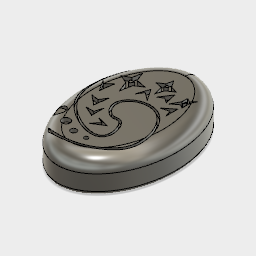
Heart of Te Fiti v12 (Autodesk Fusion 360 design; units mm, degrees)
Autodesk Fusion 360 part; units mm, degrees
sketch "Sketch1" plane through (0, 0, 0) normal (0, 1, 0) x (1, 0, 0)
  ellipse E0 centre (0, 0) end of major axis (-25.3296, 0) minor radius 36.9593
  line L0 (0, 36.9593) -> (0, -36.9593)
  spline S0 degree 5 poles (-15.7012, 29.002) (-15.9891, 28.3491) (-16.546, 27.0466) (-17.3246, 25.1025) (-18.2491, 22.5296) (-19.2149, 19.3463) (-19.9901, 16.1981) (-20.573, 13.0893) (-20.9615, 10.0271) (-21.1523, 7.0224) (-21.1416, 4.0904) (-20.9226, 1.2494) (-20.4826, -1.4829) (-19.7996, -4.0921) (-18.84, -6.57) (-17.5537, -8.9182) (-15.8765, -11.1484) (-13.7557, -13.2651) (-11.1725, -15.2534) (-8.1669, -17.0617) (-4.8575, -18.5914) (-1.4746, -19.6732) (1.6501, -20.0831) (4.1724, -19.6282) (5.8128, -18.2238) (6.4275, -15.9592) (6.1099, -13.2065) (5.1666, -10.5598) (3.9551, -8.5895) (2.7709, -7.6638) (1.6883, -7.7026) (0.4948, -8.076) (-1.034, -8.0508) (-2.8425, -7.2512) (-4.6232, -5.6824) (-5.9927, -3.5531) (-6.6094, -1.1715) (-6.3383, 1.2047) (-5.2263, 3.3819) (-3.4309, 5.2146) (-1.1685, 6.6006) (1.3532, 7.4698) (3.9703, 7.7796) (6.5518, 7.5146) (8.9989, 6.6859) (11.24, 5.3299) (13.2285, 3.5089) (14.9372, 1.306) (16.35, -1.1845) (17.4553, -3.8656) (18.2388, -6.6462) (18.6749, -9.4504) (18.7235, -12.2234) (18.3412, -14.9247) (17.4911, -17.5231) (16.1529, -19.9908) (14.3329, -22.2983) (12.0743, -24.4089) (9.4475, -26.2812) (6.5404, -27.8718) (3.4481, -29.1384) (0.2632, -30.0424) (-2.9336, -30.5517) (-6.0847, -30.6437) (-9.1516, -30.3038) (-12.1117, -29.5237) (-14.3851, -28.5443) (-16.0353, -27.6096) (-17.1111, -26.8975) (-17.6429, -26.5192) knots 0 0 0 0 0 0 0.01538462 0.03076923 0.04615385 0.06153846 0.07692308 0.09230769 0.10769231 0.12307692 0.13846154 0.15384615 0.16923077 0.18461538 0.2 0.21538462 0.23076923 0.24615385 0.26153846 0.27692308 0.29230769 0.30769231 0.32307692 0.33846154 0.35384615 0.36923077 0.38461538 0.4 0.41538462 0.43076923 0.44615385 0.46153846 0.47692308 0.49230769 0.50769231 0.52307692 0.53846154 0.55384615 0.56923077 0.58461538 0.6 0.61538462 0.63076923 0.64615385 0.66153846 0.67692308 0.69230769 0.70769231 0.72307692 0.73846154 0.75384615 0.76923077 0.78461538 0.8 0.81538462 0.83076923 0.84615385 0.86153846 0.87692308 0.89230769 0.90769231 0.92307692 0.93846154 0.95384615 0.96923077 0.98461538 1 1 1 1 1 1
  spline S1 degree 3 poles (-16.6162, 29.4055) (-19.4737, 22.9258) (-21.2452, 16.5844) (-21.871, 10.5048) (-22.3276, 6.0685) (-22.195, 1.7935) (-21.2955, -2.1346) (-20.5773, -5.2711) (-19.3583, -8.1903) (-17.2819, -10.8547) (-15.6727, -12.9195) (-13.5224, -14.8439) (-10.8813, -16.5273) (-8.5658, -18.0031) (-5.866, -19.3042) (-3.1892, -20.1044) (-0.8686, -20.7982) (1.4051, -21.1094) (3.2946, -20.663) (4.5251, -20.3723) (5.6026, -19.7124) (6.2825, -18.7299) (7.1836, -17.4276) (7.3498, -15.6939) (7.112, -14.0022) (6.8652, -12.2461) (6.209, -10.5186) (5.4431, -9.2339) (4.856, -8.2491) (4.2062, -7.505) (3.4287, -7.095) (2.8556, -6.7929) (2.2196, -6.7275) (1.7142, -6.7735) (0.9777, -6.8405) (0.4776, -7.0104) (-0.0835, -6.9994) (-0.6436, -6.9884) (-1.3083, -6.8203) (-2.0532, -6.3723) (-3.1341, -5.7222) (-4.2876, -4.4772) (-4.8945, -3.0786) (-5.5405, -1.5898) (-5.5712, -0.0001) (-4.9649, 1.4393) (-4.2274, 3.19) (-2.521, 4.7438) (-0.4724, 5.6612) (1.5863, 6.5831) (3.9224, 6.8611) (6.0735, 6.4445) (8.7058, 5.9347) (11.0949, 4.3826) (12.9846, 2.0916) (15.2894, -0.7024) (16.8696, -4.5298) (17.4301, -8.2498) (17.9455, -11.6702) (17.5729, -14.9779) (16.0429, -17.9581) (14.7902, -20.3981) (12.7277, -22.6602) (10.0863, -24.5365) (6.8505, -26.835) (2.8163, -28.5153) (-1.13, -29.199) (-4.8782, -29.8484) (-8.5276, -29.611) (-11.8947, -28.4189) (-13.6843, -27.7852) (-15.4056, -26.8835) (-17.0633, -25.7044) knots 0 0 0 0 0.09047855 0.09047855 0.09047855 0.15650286 0.15650286 0.15650286 0.20922143 0.20922143 0.20922143 0.25007582 0.25007582 0.25007582 0.28589274 0.28589274 0.28589274 0.3169454 0.3169454 0.3169454 0.3371678 0.3371678 0.3371678 0.36397047 0.36397047 0.36397047 0.39179297 0.39179297 0.39179297 0.41311949 0.41311949 0.41311949 0.42883763 0.42883763 0.42883763 0.45174167 0.45174167 0.45174167 0.47460508 0.47460508 0.47460508 0.50778137 0.50778137 0.50778137 0.54309603 0.54309603 0.54309603 0.58604666 0.58604666 0.58604666 0.62920969 0.62920969 0.62920969 0.68202832 0.68202832 0.68202832 0.7464456 0.7464456 0.7464456 0.80567522 0.80567522 0.80567522 0.85416995 0.85416995 0.85416995 0.91357908 0.91357908 0.91357908 0.97000737 0.97000737 0.97000737 1 1 1 1
  line L1 (-18.7775, -24.805) -> (-17.0633, -25.7044)
  line L2 (2, -13) -> (-3.7121, -16.5136)
  line L3 (-3.7121, -16.5136) -> (-0.856, -13)
  line L4 (-0.856, -13) -> (-3.7121, -11.6455)
  line L5 (-3.7121, -11.6455) -> (2, -13)
  line L6 (-6.8234, -12.3227) -> (-6.8234, -6)
  line L7 (-6.8234, -6) -> (-8, -10)
  line L8 (-8, -10) -> (-12, -10)
  line L9 (-12, -10) -> (-6.8234, -12.3227)
  line L10 (-16, -3) -> (-10.994, -7.0691)
  line L11 (-10.994, -7.0691) -> (-10, 0)
  line L12 (-10, 0) -> (-12.2593, -3.5345)
  line L13 (-12.2593, -3.5345) -> (-16, -3)
  line L14 (-20, 7) -> (-16, 1)
  line L15 (-16, 1) -> (-15, 8)
  line L16 (-15, 8) -> (-18, 5)
  line L17 (-18, 5) -> (-20, 7)
  line L18 (-17.1699, 13.2946) -> (-12.8176, 11.6267)
  line L19 (-12.8176, 11.6267) -> (-10.5661, 5.9978)
  line L20 (-10.5661, 5.9978) -> (-9.464, 11.8697)
  line L21 (-9.464, 11.8697) -> (-5.6699, 14.4447)
  line L22 (-5.6699, 14.4447) -> (-10.6699, 15.3832)
  line L23 (-10.6699, 15.3832) -> (-12.5397, 20.0577)
  line L24 (-12.5397, 20.0577) -> (-13.4171, 15.3832)
  line L25 (-13.4171, 15.3832) -> (-17.1699, 13.2946)
  line L26 (-12.9292, 13.9595) -> (-11.7996, 11.9649)
  line L27 (-11.7996, 11.9649) -> (-10.5246, 13.9595)
  line L28 (-10.5246, 13.9595) -> (-12.9292, 13.9595)
  line L29 (14.5337, 21.6256) -> (12.8041, 19.3149)
  line L30 (12.8041, 19.3149) -> (10.7477, 20.4148)
  line L31 (10.7477, 20.4148) -> (10.7477, 17.5434)
  line L32 (10.7477, 17.5434) -> (8.3775, 13.112)
  line L33 (8.3775, 13.112) -> (11.6761, 15.7091)
  line L34 (11.6761, 15.7091) -> (13.5759, 14.693)
  line L35 (13.5759, 14.693) -> (13.5759, 18.1878)
  line L36 (13.5759, 18.1878) -> (14.5337, 21.6256)
  line L37 (11.8441, 16.623) -> (12.6269, 18.0864)
  line L38 (12.6269, 18.0864) -> (11.8441, 18.5051)
  line L39 (11.8441, 18.5051) -> (11.8441, 16.623)
  line L40 (-5, 9) -> (-3, 15)
  line L41 (-3, 15) -> (1, 9)
  line L42 (1, 9) -> (-3, 12)
  line L43 (-3, 12) -> (-5, 9)
  line L44 (2, 13) -> (5.761, 18.6416)
  line L45 (5.761, 18.6416) -> (7, 13)
  line L46 (7, 13) -> (4.6288, 14.5808)
  line L47 (4.6288, 14.5808) -> (2, 13)
  line L48 (8, 9) -> (13, 13)
  line L49 (13, 13) -> (13, 7)
  line L50 (13, 7) -> (12, 10)
  line L51 (12, 10) -> (8, 9)
  line L52 (0, 14) -> (1.3214, 17.9641)
  line L53 (1.3214, 17.9641) -> (4.7927, 20.2783)
  line L54 (4.7927, 20.2783) -> (1.3214, 21.4354)
  line L55 (1.3214, 21.4354) -> (-0.8933, 24.7574)
  line L56 (-0.8933, 24.7574) -> (-1.5471, 21.4354)
  line L57 (-1.5471, 21.4354) -> (-4.7582, 19.2947)
  line L58 (-4.7582, 19.2947) -> (-1.2202, 18.5984)
  line L59 (-1.2202, 18.5984) -> (0, 14)
  line L60 (-0.6101, 21.4354) -> (0.6607, 20.3651)
  line L61 (0.6607, 20.3651) -> (-0.6101, 19.2947)
  line L62 (-0.6101, 19.2947) -> (-0.6101, 21.4354)
  circle A0 centre (-18.5, -17.5) radius 2.9155
  circle A1 centre (-11, -21.5) radius 2.0616
  circle A2 centre (-4.5, -24) radius 1.5
  circle A3 centre (2, -24) radius 1
  point P0 (-21, 9)
  point P1 (-19, -6)
  point P2 (-6, -18)
  point P3 (6, -17)
  point P4 (3, -8)
  point P5 (0, -8)
  point P6 (-6, -3)
  point P7 (-2, 6)
  point P8 (10, 6)
  point P9 (18, -6)
  point P10 (16, -20)
  point P11 (0, -30)
  point P12 (-18.05, 25.9294)
  point P13 (-18.6, 26.3)
  dimension "d22" = 1
sketch "Sketch6" plane through (0, 0, 0) normal (0, 1, 0) x (1, 0, 0)
  ellipse E0 centre (0, 0) end of major axis (-25.3296, 0) minor radius 36.9593
  line L0 (-15.4592, 16.8238) -> (3.0408, 16.8238)
  line L1 (3.0408, 16.8238) -> (3.0408, -16.6887)
  line L2 (3.0408, -16.6887) -> (-15.4592, -16.6887)
  line L3 (-15.4592, -16.6887) -> (-15.4592, 16.8238)
  line L4 (4, 15) -> (4, -14.5)
  line L5 (4, -14.5) -> (19.5, -14.5)
  line L6 (19.5, -14.5) -> (19.5, 15)
  line L7 (19.5, 15) -> (4, 15)
  line L8 (-16.5772, 17.6949) -> (14.4228, 17.6949)
  line L9 (14.4228, 17.6949) -> (14.4228, -17.3051)
  line L10 (14.4228, -17.3051) -> (-16.5772, -17.3051)
  line L11 (-16.5772, -17.3051) -> (-16.5772, 17.6949)
  line L12 (-23.4538, 3.2894) -> (-20.0538, 3.2894)
  line L13 (-20.0538, 3.2894) -> (-20.0538, -2.8106)
  line L14 (-20.0538, -2.8106) -> (-23.4538, -2.8106)
  line L15 (-23.4538, -2.8106) -> (-23.4538, 3.2894)
  line L16 (-14.2116, 19.8935) -> (-17.2758, 22.4647)
  line L17 (-17.2758, 22.4647) -> (-10.8479, 30.1251)
  line L18 (-10.8479, 30.1251) -> (-7.7838, 27.554)
  line L19 (-7.7838, 27.554) -> (-14.2116, 19.8935)
  line L20 (14.6302, 19.8313) -> (7.5591, 26.9024)
  line L21 (17.4586, 22.6598) -> (14.6302, 19.8313)
  line L22 (7.5591, 26.9024) -> (10.3876, 29.7308)
  line L23 (10.3876, 29.7308) -> (17.4586, 22.6598)
  line L24 (-24.4399, -1.508) -> (-24.4399, 1.992)
  line L25 (-24.4399, 1.992) -> (-22.5353, 14.9175)
  line L26 (-22.5353, 14.9175) -> (-20, 14.9175)
  line L27 (-20, 14.9175) -> (-23.4538, 3.2894)
  line L28 (-24.4399, -1.508) -> (-23, -14)
  line L29 (-12.212, -23.2906) -> (-4.5516, -29.7185)
  line L30 (-14.7831, -26.3548) -> (-12.212, -23.2906)
  line L31 (-4.5516, -29.7185) -> (-7.1227, -32.7827)
  line L32 (-7.1227, -32.7827) -> (-14.7831, -26.3548)
  line L33 (7.0782, -33.2768) -> (4.5071, -30.2126)
  line L34 (14.7387, -26.8489) -> (7.0782, -33.2768)
  line L35 (12.1675, -23.7847) -> (14.7387, -26.8489)
  line L36 (4.5071, -30.2126) -> (12.1675, -23.7847)
  line L37 (20.1173, 4.5042) -> (24.1173, 4.5042)
  line L38 (24.1173, 4.5042) -> (24.1173, -5.4958)
  line L39 (24.1173, -5.4958) -> (20.1173, -5.4958)
  line L40 (20.1173, -5.4958) -> (20.1173, 4.5042)
  line L41 (-20.0538, 3.2894) -> (-20, 14.9175)
  line L42 (-20.0538, 4.1184) -> (-15.4592, 5.3136)
  line L43 (-10.3194, -24.8787) -> (-8.4193, -16.6887)
  line L44 (-7.1227, -27.5611) -> (-4.6002, -16.6887)
  line L45 (9.7896, -25.78) -> (0.2605, -16.6887)
  line L46 (-12.0492, 22.4706) -> (-11.4924, 16.8238)
  line L47 (-9.5498, 25.4493) -> (-8.6994, 16.8238)
  line L48 (9.6455, 24.816) -> (-4.9023, 16.8238)
  line L49 (11.9074, 22.5541) -> (1.4768, 16.8238)
  line L50 (20.1173, 1.1648) -> (19.5, 1.1648)
  line L51 (19.5, -1.7393) -> (20.1173, -1.7393)
  line L52 (3.0408, 1.8565) -> (4, 1.8565)
  line L53 (3.0408, -1.3066) -> (4, -1.3066)
  line L54 (-23, -14) -> (-20, -14)
  line L55 (-20, -14) -> (-23.4538, -2.8106)
  line L56 (-20.0538, -2.8106) -> (-20, -14)
  line L57 (-20.0504, -3.5272) -> (-15.4592, -4.5753)
  line L58 (7.038, -28.0889) -> (-3.1314, -16.6887)
  line L59 (-20.0538, 2.2355) -> (-17.5, 2.2355)
  line L60 (-17.5, 2.2355) -> (-17.5, -1.779)
  line L61 (-17.5, -1.779) -> (-20.0538, -1.779)
  line L62 (-24.4399, 1.992) -> (-23.4538, 1.992)
  line L63 (-24.4399, -1.508) -> (-23.4538, -1.508)
  dimension "d29" = 35
  dimension "d30" = 31
  dimension "d31" = 3.4
  dimension "d32" = 6.1
  dimension "d33" = 10
  dimension "d34" = 4
  dimension "d35" = 10
  dimension "d36" = 4
  dimension "d38" = 3.5
  dimension "d40" = 10
  dimension "d41" = 4
  dimension "d42" = 10
  dimension "d43" = 4
  dimension "d46" = 4
  dimension "d47" = 10
  measures "d29" distance of L8.start L10.end
  measures "d30" distance of L8.start L8.end
  measures "d31" distance of L12.start L12.end
  measures "d32" distance of L12.start L14.end
  measures "d33" distance of L16.start L18.end
  measures "d34" distance of L16.start L16.end
  measures "d35" distance of L20.start L20.end
  measures "d36" distance of L20.end L22.end
  measures "d38" distance of L24.end L24.start
  measures "d40" distance of L31.end L30.start
  measures "d41" distance of L30.start L29.start
  measures "d42" distance of L33.end L35.start
  measures "d43" distance of L35.start L34.start
  measures "d46" distance of L37.start L37.end
  measures "d47" distance of L37.start L39.end
extrude "Extrude12" add sketch "Sketch6" along normal blind 5 contours E0 | L0 L3 L8 L11 L42 L46 | L0 L1 L2 L3 | L0 L8 L46 L47 | L3 L11 L42 L57 | L0 L8 L47 L48 | L8 L19 L46 L47 | L2 L3 L10 L11 L43 L57 | L11 L13 L41 L42 L56 L57 L59 L60 L61 | L0 L8 L48 L49 | L16 L17 L18 L19 | L12 L27 L41 | L0 L1 L4 L7 L8 L9 L49 L52 | L8 L20 L48 L49 | L2 L10 L43 L44 | L14 L55 L56 | L12 L13 L14 L15 | L15 L25 L26 L27 L62 | L20 L21 L22 L23 | L2 L10 L44 L58 | L10 L29 L43 L44 | L15 L28 L54 L55 L63 | L13 L59 L60 L61 | L1 L4 L52 L53 | L2 L10 L45 L58 | L29 L30 L31 L32 | L15 L24 L62 L63 | L1 L2 L4 L5 L9 L10 L45 L53 | L4 L5 L7 L9 | L5 L6 L7 L9 | L10 L36 L45 L58 | L33 L34 L35 L36 | L6 L40 L50 L51 | L37 L38 L39 L40 makes body 1
move_face "MoveFace1" to x (1, 0, 0) y (0, 1, 0) z (0, 0, 1) at (0, 10, 0) 1 faces at (-25.2434, 3.3333, -3.0473) on bodies 1
extrude "Extrude17" add sketch "Sketch6" along normal blind 5 separate body contours E0 | L0 L3 L8 L11 L42 L46 | L0 L8 L47 L48 | L2 L3 L10 L11 L43 L57 | L12 L27 L41 | L0 L1 L4 L7 L8 L9 L49 L52 | L14 L55 L56 | L2 L10 L44 L58 | L13 L59 L60 L61 | L1 L2 L4 L5 L9 L10 L45 L53 makes body 2 at (-17.5, 1.6667, -0.8973) makes body 3 at (-1.709, 0, -23.7601)
extrude "Extrude18" add sketch "Sketch6" along normal blind 5 separate body contours E0 | L12 L27 L41 | L14 L55 L56 | L13 L59 L60 L61 makes body 4 at (-17.5, 1.6667, -0.8973) makes body 5 at (0.1416, 0, -30.4678)
move_body "Move5" bodies 1 to x (1, 0, 0) y (0, 1, 0) z (0, 0, 1) at (0, 10, 0)
move_body "Move6" bodies 2 3 to x (1, 0, 0) y (0, 1, 0) z (0, 0, 1) at (0, 5, 0)
combine "Combine6" operation add target body 1 tool bodies 4 2 3 5
fillet "Fillet3" radius 7 1 edges at (0, 15, -36.9593) on bodies 1
extrude "Extrude19" add sketch "Sketch1" along normal blind 4 separate body contours E0 L0 S0 S1 L1 | L0 S0 S1 | E0 L0 S0 S1 | L0 L52 L53 L54 L55 L60 L61 | L0 L55 L56 L57 L58 L59 L60 L61 L62 | L0 S0 S1 | L0 S0 S1 | L0 L40 L41 L42 L43 | L0 L41 L42 | L0 L2 L3 L4 L5 | L0 L2 L5 | L6 L7 L8 L9 | L10 L11 L12 L13 | L14 L15 L16 L17 | L18 L19 L20 L21 L22 L23 L24 L25 | L29 L30 L31 L32 L33 L34 L35 L36 | L44 L45 L46 L47 | L48 L49 L50 L51 | A0 | A1 | A2 | A3 makes body 6 at (-3.0019, 2.6667, 24.0748) makes body 7 at (-6.8234, 1.3333, 10.2152) makes body 8 at (9.9576, 1.3333, -16.0662) makes body 9 at (-12.2089, 0, -16.9413) makes body 10 at (3.2537, 1.3333, -14.8805) makes body 11 at (-10.6627, 1.3333, 4.7127) makes body 12 at (1.3018, 2.6667, 24.7159) makes body 13 at (-8.941, 2.6667, 21.6028) makes body 14 at (-20.3172, 2.6667, -14.3248) makes body 15 at (9.6667, 1.3333, -10.3333) makes body 16 at (-1.6667, 1.3333, -13) makes body 17 at (-2.5085, 0, -19.7762) makes body 18 at (-18.6667, 1.3333, -5) makes body 19 at (-1.808, 1.3333, 15.3424) makes body 20 at (-15.5881, 2.6667, 17.6453)
move_body "Move7" bodies 6 19 20 17 18 15 8 16 13 14 12 10 11 7 9 to x (1, 0, 0) y (0, 1, 0) z (0, 0, 1) at (0, 8, 0)
move_body "Move8" bodies 6 19 20 17 18 15 8 16 13 14 12 10 11 7 9 to x (1, 0, 0) y (0, 1, 0) z (0, 0, 1) at (0, 5, 0)
combine "Combine7" operation cut target body 1 tool bodies 6 19 20 17 18 15 8 16 13 14 12 10 11 7 9
extrude "Extrude20" add sketch "Sketch6" along normal blind 5 separate body contours L12 L13 L14 L15 makes body 21
move_body "Move9" bodies 21 to x (1, 0, 0) y (0, 1, 0) z (0, 0, 1) at (0, 5, 0)
combine "Combine8" operation add target body 1 tool bodies 21
extrude "Extrude21" add sketch "Sketch6" along normal blind 2 separate body contours E0 | L0 L3 L8 L11 L42 L46 | L0 L1 L2 L3 | L0 L8 L46 L47 | L3 L11 L42 L57 | L0 L8 L47 L48 | L8 L19 L46 L47 | L2 L3 L10 L11 L43 L57 | L11 L13 L41 L42 L56 L57 L59 L60 L61 | L0 L8 L48 L49 | L16 L17 L18 L19 | L12 L27 L41 | L0 L1 L4 L7 L8 L9 L49 L52 | L8 L20 L48 L49 | L2 L10 L43 L44 | L14 L55 L56 | L12 L13 L14 L15 | L15 L25 L26 L27 L62 | L20 L21 L22 L23 | L2 L10 L44 L58 | L10 L29 L43 L44 | L15 L28 L54 L55 L63 | L13 L59 L60 L61 | L1 L4 L52 L53 | L2 L10 L45 L58 | L29 L30 L31 L32 | L15 L24 L62 L63 | L1 L2 L4 L5 L9 L10 L45 L53 | L4 L5 L7 L9 | L5 L6 L7 L9 | L10 L36 L45 L58 | L33 L34 L35 L36 | L6 L40 L50 L51 | L37 L38 L39 L40 makes body 22
move_body "Move10" bodies 22 to x (1, 0, 0) y (0, 1, 0) z (0, 0, 1) at (0, -2, 0)
fillet "Fillet4" radius 2 1 edges at (0, -2, -36.9593) on bodies 22
hole "Hole1" at (-0.5262, -2, 26.1547) direction (0, 1, 0) diameter 2 depth 6 tip angle 180 countersink diameter 2.5 countersink angle 90 bodies 1 22
hole "Hole2" at (-3.4733, -2, -26.1776) direction (0, 1, 0) diameter 2 depth 6 tip angle 180 countersink diameter 2.5 countersink angle 90 bodies 1 22
named bodies: "Heart", "Cover"
